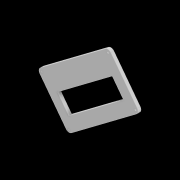
# Autodesk Inventor part: switchback-osc-cover
Saved by Autodesk Inventor 2020 (Build 240168000, 168)
## iProperties
Created: 2020-01-13
Part Number: switchback-osc-cover
Material: Generic
Document SubType Name: Modeling
Designer: valer
Density: 1 g/cm^3
Appearance: Default
Author: valer
Autodesk Inventor part; units mm, degrees
ref_plane "YZ Plane" through (0, 0, 0) normal (1, 0, 0) x (0, 1, 0)
ref_plane "XZ Plane" through (0, 0, 0) normal (0, 1, 0) x (-1, 0, 0)
ref_plane "XY Plane" through (0, 0, 0) normal (0, 0, 1) x (1, 0, 0)
sketch "Profile" plane through (0, 0, 0) normal (0, 0, 1) x (1, 0, 0)
  line L0 (40.533, 3.3564) -> (-14.4186, -37.9517)
  arc A0 (-18.8598, -37.3276) -> (-14.4186, -37.9517) centre (-16.3264, -35.4138) ccw
  line L1 (-18.8598, -37.3276) -> (-41.1587, -7.8081)
  arc A1 (-40.533, -3.3564) -> (-41.1587, -7.8081) centre (-38.6253, -5.8943) ccw
  line L2 (-40.533, -3.3564) -> (14.4186, 37.9517)
  arc A2 (18.8598, 37.3276) -> (14.4186, 37.9517) centre (16.3264, 35.4138) ccw
  line L3 (18.8598, 37.3276) -> (41.1587, 7.8081)
  arc A3 (40.533, 3.3564) -> (41.1587, 7.8081) centre (38.6253, 5.8943) ccw
  circle A4 centre (39.6613, 5.7487) radius 0.635
  circle A5 centre (-16.5289, -36.8546) radius 0.635
  circle A6 centre (-39.5611, -5.7628) radius 0.635
  circle A7 centre (16.4321, 36.166) radius 0.635
  line L4 (29.3865, 8.0454) -> (-16.5242, -26.4666)
  arc A8 (-16.8798, -26.4161) -> (-16.5242, -26.4666) centre (-16.6768, -26.2635) ccw
  line L5 (-16.8798, -26.4161) -> (-26.1135, -14.1327)
  arc A9 (-26.0631, -13.777) -> (-26.1135, -14.1327) centre (-25.9105, -13.9801) ccw
  line L6 (-26.0631, -13.777) -> (19.8476, 20.7349)
  arc A10 (20.2032, 20.6845) -> (19.8476, 20.7349) centre (20.0002, 20.5319) ccw
  line L7 (20.2032, 20.6845) -> (29.4369, 8.401)
  arc A11 (29.3865, 8.0454) -> (29.4369, 8.401) centre (29.2339, 8.2484) ccw
  point P0 (0, 0)
  constraints: 16 end point, 16 point on circle, 12 centre point
extrude "BaseFeature" add sketch "Profile" along normal blind 2.54
body "Solid1"
